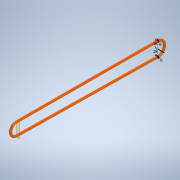
# Autodesk Inventor part: RoundBelt
Saved by Autodesk Inventor 2021 (Build 250183000, 183)
## iProperties
Created: 2021-05-22
Part Number: RoundBelt
Material: PAEK Plastic
Document SubType Name: Modeling
Designer: sami8
Density: 1.32 g/cm^3
Appearance: Smooth - Light Orange
Author: sami8
Autodesk Inventor part; units mm, degrees
ref_plane "YZ Plane" through (0, 0, 0) normal (1, 0, 0) x (0, 1, 0)
ref_plane "XZ Plane" through (0, 0, 0) normal (0, 1, 0) x (-1, 0, 0)
sketch "Sketch1" plane through (0, 0, 0) normal (0, 0, 1) x (1, 0, 0)
  line L0 (0, 0) -> (17.1365, 0)
  line L1 (0, 0) -> (0, 18) construction
  line L2 (0, 0) -> (0, -18) construction
  circle A0 centre (0, 18) radius 3
  circle A1 centre (0, -18) radius 3
  dimension "d0" = 18
  dimension "d1" = 18
  dimension "d2" = 6
  dimension "d3" = 6
  constraints: 6 end point, 2 centre point, 2 coincident, 2 vertical, 1 horizontal
  measures "d0" distance of L0.start L1.end
  measures "d1" distance of L0.start L2.end
  measures "d2" diameter of A0
  measures "d3" diameter of A1
ref_plane "Work Plane1" through (0, 0, 365.4) normal (0, 0, 1) x (1, 0, 0)
sketch "Sketch3" plane through (0, 0, 365.4) normal (0, 0, 1) x (1, 0, 0)
  line L0 (-3.5, 0) -> (-3.5, 15.9) construction
  line L1 (-3.5, 0) -> (-3.5, -15.9) construction
  circle A0 centre (-3.5, 15.9) radius 3
  circle A1 centre (-3.5, -15.9) radius 3
  line L2 (0, 0) -> (-3.5, 0)
  dimension "d8" = 15.9
  dimension "d9" = 15.9
  dimension "d10" = 6
  dimension "d11" = 6
  dimension "d17" = 3.5
  constraints: 6 end point, 2 centre point, 2 coincident, 2 vertical, 1 horizontal
  measures "d8" distance of L0.start L0.end
  measures "d9" distance of L0.start L1.end
  measures "d10" diameter of A0
  measures "d11" diameter of A1
  measures "d17" distance of L2.start L0.start
revolve "Revolution1" add sketch "Sketch1" angle 180 about axis through (0, 0, 0) along (-1, 0, 0) contours A0
sketch3d "3D Sketch1"
  line L0 (-3.5, 15.9, 365.4) -> (0, 18, 0)
sweep "Sweep1" add profiles "Sketch3" path "3D Sketch1" contours A0
sketch3d "3D Sketch1 for Sweep2"
  line L0 (-3.5, -15.9, 365.4) -> (0, -18, 0)
sweep "Sweep2" add profiles "Sketch3" path "3D Sketch1 for Sweep2" contours A1
revolve "Revolution2" add sketch "Sketch3" angle 180 about axis through (0, 0, 365.4) along (1, 0, 0) contours A0
equation "\"d8\" = d9"
body "Solid1"
